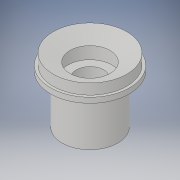
# Autodesk Inventor part: Phenlic
Saved by Autodesk Inventor 2017 (Build 210142000, 142)
## iProperties
Created: 2016-07-19
Part Number: Phenlic
Material: Generic
Document SubType Name: Modeling
Designer: Bill
Density: 1 g/cm^3
Appearance: Default
Author: Bill
Autodesk Inventor part; units mm, degrees
ref_plane "YZ Plane" through (0, 0, 0) normal (1, 0, 0) x (0, 1, 0)
ref_plane "XZ Plane" through (0, 0, 0) normal (0, 1, 0) x (-1, 0, 0)
ref_plane "XY Plane" through (0, 0, 0) normal (0, 0, 1) x (1, 0, 0)
sketch "Sketch1" plane through (0, 0, 0) normal (0, 0, 1) x (1, 0, 0)
  line L0 (-67.183, -7.8688) -> (-67.183, 109.1349)
  line L1 (-67.183, -7.8688) -> (-60.833, -7.8688)
  line L2 (-67.183, 109.1349) -> (-95.25, 109.1349)
  line L3 (-95.25, 109.1349) -> (-95.25, 121.8349)
  line L4 (-95.25, 121.8349) -> (-88.9, 121.8349)
  line L5 (-88.9, 121.8349) -> (-88.9, 147.2349)
  line L6 (-88.9, 147.2349) -> (-38.3236, 147.2349) construction
  line L7 (-60.833, -7.8688) -> (-33.1797, 95.3346)
  line L8 (-33.1797, 95.3346) -> (-53.4136, 95.3346)
  line L9 (0, -38.8896) -> (0, 178.2557) projected
  line L10 (-88.9, 147.2349) -> (-48.411, 128.3546)
  line L11 (-48.411, 128.3546) -> (-53.4136, 128.3546)
  line L12 (-53.4136, 128.3546) -> (-53.4136, 95.3346)
  point P0 (0, 0)
  dimension "d0" = 6.35
  dimension "d1" = 60.833
  dimension "d4" = 12.7
  dimension "d5" = 28.067
  dimension "d6" = 25.4
  dimension "d9" = 6.35
  dimension "d10" = 105
  dimension "d16" = 20.2339
  dimension "d17" = 25
  dimension "d18" = 5.0026
  dimension "d19" = 33.02
  dimension "d20" = 33.1797
  dimension "d21" = 95.25
  dimension "d22" = 117.0038
  constraints: 24 end point, 6 horizontal, 3 perpendicular, 1 vertical
  measures "d0" distance of L0.start L1.end
  measures "d1" horizontal distance of point (0, 0) L1.end
  measures "d4" distance of L2.end L3.end
  measures "d5" distance of L0.end L2.end
  measures "d6" distance of L4.end L5.end
  measures "d9" distance of L3.end L4.end
  measures "d10" angle of L1 L7
  measures "d16" distance of L7.end L8.end
  measures "d17" angle of L6 L10
  measures "d18" distance of L10.end L11.end
  measures "d19" distance of L11.end L8.end
  measures "d20" distance from line of L9 L7.end
  measures "d21" distance between parallel lines of L9 L3
  measures "d22" distance of L0.start L0.end
revolve "Revolution1" add sketch "Sketch1" angle 360 about axis through (0, -10, 0) along (0, 1, 0)
body "Solid1"
